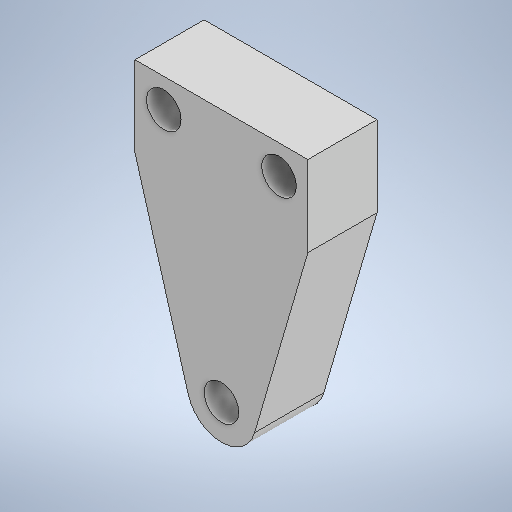
# Autodesk Inventor part: SteeringBase
Saved by Autodesk Inventor 2025.2 (Build 292293000, 293)
## iProperties
Created: 2025-01-08
Part Number: SteeringBase
Material: 일반
Document SubType Name: Modeling
Designer: SEON
Density: 1 g/cm^3
Appearance: 기본값
Author: SEON
Autodesk Inventor part; units mm, degrees
ref_plane "YZ Plane" through (0, 0, 0) normal (1, 0, 0) x (0, 1, 0)
ref_plane "XZ Plane" through (0, 0, 0) normal (0, 1, 0) x (-1, 0, 0)
ref_plane "XY Plane" through (0, 0, 0) normal (0, 0, 1) x (1, 0, 0)
sketch "스케치1" plane through (0, 0, 0) normal (0, 0, 1) x (1, 0, 0)
  circle A0 centre (0, 0) radius 1.5
  arc A1 (-2.88, -0.84) -> (2.88, -0.84) centre (0, 0) ccw
  line L0 (-7.5, 22) -> (7.5, 22)
  line L1 (7.5, 22) -> (7.5, 15)
  line L2 (-7.5, 15) -> (-7.5, 22)
  line L3 (-7.5, 15) -> (-2.88, -0.84)
  line L4 (7.5, 15) -> (2.88, -0.84)
  circle A2 centre (-5, 19.5) radius 1.5
  circle A3 centre (5, 19.5) radius 1.5
  point P0 (0, 22)
  point P1 (0, -3)
  dimension "d0" = 3
  dimension "d1" = 6
  dimension "d2" = 3
  dimension "d3" = 3
  dimension "d4" = 15
  dimension "d5" = 25
  dimension "d6" = 2.5
  dimension "d7" = 2.5
  dimension "d8" = 2.5
  dimension "d9" = 7
  constraints: 10 end point, 4 centre point, 3 point on circle, 2 coincident, 2 horizontal alignment, 2 tangent, 1 horizontal, 1 midpoint, 1 parallel, 1 perpendicular, 1 vertical alignment
  measures "d0" diameter of A0
  measures "d1" diameter of A1
  measures "d2" diameter of A2
  measures "d3" diameter of A3
  measures "d4" distance of L0.start L0.end
  measures "d5" distance from line of point (0, -3) L0
  measures "d6" distance from line of L0 A2.centre
  measures "d7" distance from line of L2 A2.centre
  measures "d8" distance from line of L1 A3.centre
  measures "d9" distance from line of L0 L2.start
extrude "돌출1" add sketch "스케치1" along normal blind 6
equation "\"d7\" = d6"
equation "\"d8\" = d7"
